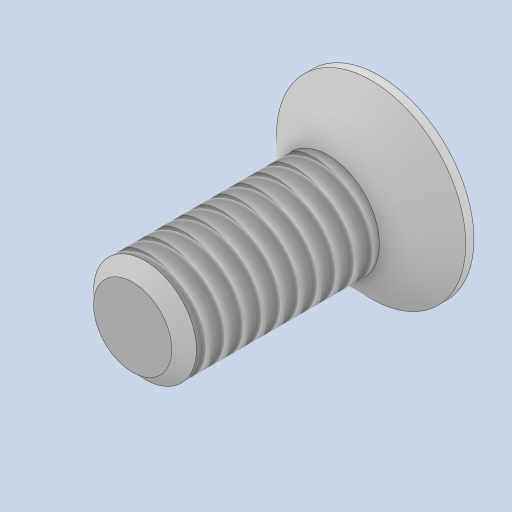
# Autodesk Inventor part: CSHCS-SUS-M2_5-6
Saved by Autodesk Inventor 2023 (Build 270158000, 158)
## iProperties
Created: 2024-12-12
Part Number: CSHCS-SUS-M2_5-6
Material: Generic
Document SubType Name: Modeling
Designer: kiyo
Density: 1 g/cm^3
Appearance: Default
Author: kiyo
Autodesk Inventor part; units mm, degrees
ref_plane "YZ Plane" through (0, 0, 0) normal (1, 0, 0) x (0, 1, 0)
ref_plane "XZ Plane" through (0, 0, 0) normal (0, 1, 0) x (-1, 0, 0)
ref_plane "XY Plane" through (0, 0, 0) normal (0, 0, 1) x (1, 0, 0)
sketch "スケッチ1" plane through (0, 0, 0) normal (0, 1, 0) x (-1, 0, 0)
  line L0 (0, 0) -> (4.75, 0)
  line L1 (4.75, 0) -> (4.75, 1.25)
  line L2 (0, 0.95) -> (0, 0)
  line L3 (5.8, 2.3) -> (6, 2.3)
  line L4 (6, 2.3) -> (6, 0)
  line L5 (6, 0) -> (4.75, 0)
  line L6 (4.75, 1.25) -> (0.3, 1.25)
  line L7 (0.3, 1.25) -> (0, 0.95)
  line L8 (4.75, 1.25) -> (5.8, 2.3)
  line L9 (5.8, 2.3) -> (6, 2.3)
  point P0 (6, 1.15)
  dimension "d1" = 6
  dimension "d4" = 45
  dimension "d5" = 1.25
  dimension "d6" = 0.3
  dimension "d8" = 45
  dimension "d9" = 0.2
  dimension "d10" = 1.25
  constraints: 21 end point, 4 horizontal, 2 perpendicular, 1 collinear, 1 midpoint, 1 parallel
  measures "d1" distance between parallel lines of L2 L4
  measures "d4" angle of L2 L7
  measures "d5" distance between parallel lines of L0 L6
  measures "d6" horizontal distance of L6.end L2.start
  measures "d8" angle of L5 L8
  measures "d9" distance of L3.start L3.end
  measures "d10" distance from line of point (6, 1.15) L1
revolve "回転1" add sketch "スケッチ1" angle 360 about axis through (0, 0, 0) along (-1, 0, 0)
sketch "スケッチ2" plane through (-6, 0, 0) normal (-1, 0, 0) x (0, 0, 1)
  circle A0 centre (0, 0) radius 0.95 projected
  line L0 (0, 0.8949) -> (0.775, 0.4474)
  line L1 (0.775, 0.4474) -> (0.775, -0.4474)
  line L2 (0.775, -0.4474) -> (0, -0.8949)
  line L3 (0, -0.8949) -> (-0.775, -0.4474)
  line L4 (-0.775, -0.4474) -> (-0.775, 0.4474)
  line L5 (-0.775, 0.4474) -> (0, 0.8949)
  point P0 (0, 0)
  dimension "d12" = 1.55
  constraints: 12 end point, 1 coincident, 13 other
  measures "d12" distance between parallel lines of L5 L2
extrude "押し出し1" cut sketch "スケッチ2" against normal blind 0.7 contours L0 L1 L2 L3 L4 L5
thread "ねじ1" size "M2.5x0.45" class "6g" standard "ANSI Metric M Profile" length 7.0626
